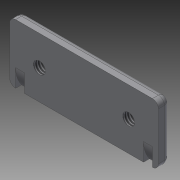
# Autodesk Inventor part: CableHolder02
Saved by Autodesk Inventor 2013 (Build 170138000, 138)
## iProperties
Created: 2013-11-09
Part Number: CableHolder02
Material: Generic
Document SubType Name: Modeling
Designer: JustinIndra
Density: 1 g/cm^3
Author: JustinIndra
Autodesk Inventor part; units mm, degrees
ref_plane "YZ Plane" through (0, 0, 0) normal (1, 0, 0) x (0, 1, 0)
ref_plane "XZ Plane" through (0, 0, 0) normal (0, 1, 0) x (-1, 0, 0)
ref_plane "XY Plane" through (0, 0, 0) normal (0, 0, 1) x (1, 0, 0)
sketch "Sketch1" plane through (0, 0, 0) normal (0, 1, 0) x (-1, 0, 0)
  line L0 (12.5, -5) -> (-12.5, -5)
  line L1 (-12.5, -5) -> (-12.5, 5)
  line L2 (-12.5, 5) -> (12.5, 5)
  line L3 (12.5, 5) -> (12.5, -5)
  point P0 (0, 0)
  point P1 (12.5, 0)
  point P2 (0, -5)
  dimension "d0" = 10
  dimension "d2" = 25
  constraints: 8 end point, 2 midpoint, 2 parallel, 1 horizontal, 1 horizontal alignment, 1 perpendicular, 1 vertical alignment
  measures "d0" distance of L2.end L0.start
  measures "d2" distance of L1.end L2.end
extrude "Extrusion1" add sketch "Sketch1" along normal blind 2
sketch "Sketch2" plane through (0, 2, 0) normal (0, 1, 0) x (1, 0, 0)
  line L0 (12.5, 5) -> (-12.5, 5) projected
  line L1 (-12.5, 5) -> (-12.5, -5) projected
  line L2 (-12.5, -5) -> (12.5, -5) projected
  line L3 (0, 5) -> (0, -5) construction
  point P0 (0, 0)
  point P1 (-7.5, 0)
  point P2 (7.5, 0)
  point P3 (0, 0)
  dimension "d5" = 5
  constraints: 3 midpoint, 2 end point, 1 horizontal alignment, 1 symmetric about line
  measures "d5" distance from line of L1 point (-7.5, 0)
hole "Hole1" at (-7.5, 2, 0) at (7.5, 2, 0) direction (0, -1, 0) diameter 2.013 end through all thread size "M2.5x0.45" class "6H" standard "ISO Metric profile"
ref_plane "Work Plane1" through (0, 5, 0) normal (0, -1, 0) x (1, 0, 0)
sketch "Sketch4" plane through (0, 5, 0) normal (0, -1, 0) x (1, 0, 0)
  line L0 (-11.5, -7) -> (-10, -7) construction
  line L1 (-10, -7) -> (-10, -2) construction
  line L2 (-10, -2) -> (-11.5, -2) construction
  line L3 (-11.5, -2) -> (-11.5, -7) construction
  line L4 (-11.5, -7) -> (-10, -7)
  line L5 (-10, -7) -> (-10, -12)
  line L6 (-10, -12) -> (-11.5, -12)
  line L7 (-11.5, -12) -> (-11.5, -7)
  line L8 (12.5, -5) -> (-12.5, -5) projected
  line L9 (-12.5, -5) -> (-12.5, 5) projected
  line L10 (-12.5, -2) -> (-10, -2)
  point P0 (0, 0)
  dimension "d15" = 3
  dimension "d16" = 5
  dimension "d17" = 5
  dimension "d18" = 1.5
  dimension "d19" = 1
  constraints: 18 end point, 4 parallel, 3 perpendicular, 2 horizontal, 1 collinear, 1 point on line
  measures "d15" distance between parallel lines of L2 L8
  measures "d16" distance of L2.end L0.start
  measures "d17" distance of L6.end L0.start
  measures "d18" distance of L0.start L0.end
  measures "d19" distance between parallel lines of L3 L9
revolve "Revolution1" cut sketch "Sketch4" angle 90 about axis through (-12.5, 5, -2) along (-1, 0, 0)
fillet "Fillet1" radius 1 8 edges at (0, 2, 5) (12.5, 1, 5) (-12.5, 1, 5) (12.5, 2, 0) (-12.5, 2, 0) (0, 2, -5) (-12.5, 1, -5) (12.5, 1, -5)
mirror "Mirror1" about plane through (0, 0, 0) normal (1, 0, 0) of "Revolution1"
body "Solid1"
